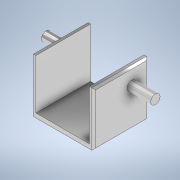
# Autodesk Inventor part: McCrea_arm-connector_Walle
Saved by Autodesk Inventor 2022 (Build 260153000, 153)
## iProperties
Created: 2022-01-26
Part Number: McCrea_arm-connector_Walle
Material: Generic
Document SubType Name: Modeling
Designer: Lukas
Density: 1 g/cm^3
Appearance: Chrome - Polished
Author: Lukas
Autodesk Inventor part; units mm, degrees
ref_plane "YZ Plane" through (0, 0, 0) normal (1, 0, 0) x (0, 1, 0)
ref_plane "XZ Plane" through (0, 0, 0) normal (0, 1, 0) x (-1, 0, 0)
ref_plane "XY Plane" through (0, 0, 0) normal (0, 0, 1) x (1, 0, 0)
sketch "Sketch1" plane through (0, 0, 0) normal (0, 1, 0) x (-1, 0, 0)
  circle A0 centre (0, 0) radius 2.2
  dimension "d0" = 4.4
  constraints: 1 centre point, 1 coincident
  measures "d0" diameter of A0
extrude "Extrusion1" add sketch "Sketch1" along normal blind 1
sketch "Sketch2" plane through (0, 1, 0) normal (0, 1, 0) x (1, 0, 0)
  line L0 (5, -6.6) -> (-5, -6.6)
  line L1 (-5, -6.6) -> (-5, 2.2)
  line L2 (-5, 2.2) -> (5, 2.2)
  line L3 (5, 2.2) -> (5, -6.6)
  circle A0 centre (0, 0) radius 2.2 projected
  line L4 (5, -6.6) -> (-5, 2.2) construction
  line L5 (-5, -6.6) -> (5, 2.2) construction
  point P0 (0, -2.2)
  dimension "d3" = 10
  constraints: 12 end point, 2 midpoint, 2 parallel, 1 horizontal, 1 perpendicular, 1 vertical alignment, 1 other
  measures "d3" distance of L0.start L0.end
extrude "Extrusion2" add sketch "Sketch2" along normal blind 0.7 contours A0 | L0 L1 L2 L3
sketch "Sketch3" plane through (0, 1.7, 0) normal (0, 1, 0) x (1, 0, 0)
  line L0 (-5, -6.6) -> (5, -6.6) projected
  line L1 (5, 2.2) -> (-5, 2.2) projected
  line L2 (-5, -6.6) -> (-4.3, -6.6)
  line L3 (-4.3, -6.6) -> (-4.3, 2.2)
  line L4 (-4.3, 2.2) -> (-5, 2.2)
  line L5 (-5, 2.2) -> (-5, -6.6)
  line L6 (5, 2.2) -> (4.3, 2.2)
  line L7 (4.3, 2.2) -> (4.3, -6.6)
  line L8 (4.3, -6.6) -> (5, -6.6)
  line L9 (5, -6.6) -> (5, 2.2)
  point P0 (0, 0)
  dimension "d6" = 0.7
  dimension "d7" = 0.7
  constraints: 16 end point, 4 parallel, 2 horizontal, 2 perpendicular, 2 point on line
  measures "d6" distance of L4.end L3.end
  measures "d7" distance of L8.end L7.end
extrude "Extrusion3" add sketch "Sketch3" along normal blind 8 contours L5 L1 L3 L0 | L7 L1 L9 L0
chamfer "Chamfer1" distance 0.3 angle 45 8 edges at (-5, 9.7, 2.2) (-5, 5.35, -2.2) (-5, 5.35, 6.6) (5, 9.7, 2.2) (5, 5.35, -2.2) (5, 5.35, 6.6) (5, 1, 2.2) (-5, 1, 2.2)
sketch "Sketch7" plane through (-5, 1.3, 6.3) normal (-1, 0, 0) x (0, 0, 1)
  line L0 (0, 0) -> (0, 8.1) projected
  line L1 (-8.2, 0) -> (0, 0) projected
  line L2 (0, 8.1) -> (-8.2, 0)
  line L3 (-8.2, 8.1) -> (-8.2, 0) projected
  line L4 (-4.1, 4.05) -> (-8.2, 4.05)
  line L5 (-8.2, 4.05) -> (-8.2, 8.1)
  line L6 (-8.2, 8.1) -> (-4.1, 8.1)
  line L7 (-4.1, 8.1) -> (-4.1, 4.05)
  line L8 (-4.1, 4.05) -> (-8.2, 4.05)
  line L9 (-8.2, 4.05) -> (-8.2, 7.55)
  line L10 (-8.2, 7.55) -> (-4.1, 7.55)
  line L11 (-4.1, 7.55) -> (-4.1, 4.05)
  circle A0 centre (-5.8287, 5.8) radius 0.75
  point P0 (-6.3, -1.3)
  dimension "d22" = 4.1
  dimension "d23" = 3.5
  dimension "d24" = 1.5
  constraints: 18 end point, 4 parallel, 2 horizontal, 2 perpendicular, 1 centre point, 1 midpoint
  measures "d22" distance of L9.end L10.end
  measures "d23" distance of L8.end L9.end
  measures "d24" diameter of A0
sketch "Sketch8" plane through (-5, 1.3, 6.3) normal (-1, 0, 0) x (0, 0, 1)
  point P0 (-6.3, -1.3)
extrude "Extrusion6" add sketch "Sketch7" along normal blind 3.8 contours A0
sketch "Sketch9" plane through (5, 1.3, -1.9) normal (1, 0, 0) x (0, 0, -1)
  circle A0 centre (-2.3713, 5.8) radius 0.75 projected
  circle A1 centre (-2.3713, 5.8) radius 0.75
  point P0 (-1.9, -1.3)
  constraints: 1 centre point, 1 coincident
extrude "Extrusion7" add sketch "Sketch9" along normal blind 3.8
body "Solid1"
